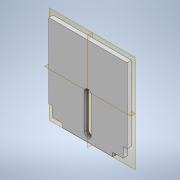
# Autodesk Inventor part: Hammer_wall
Saved by Autodesk Inventor 2021 (Build 250183000, 183)
## iProperties
Created: 2021-02-17
Part Number: Hammer_wall
Material: Generic
Document SubType Name: Modeling
Designer: negt20
Density: 1 g/cm^3
Appearance: Default
Author: negt20
Autodesk Inventor part; units mm, degrees
sketch "Sketch1" plane through (0, 0, 0) normal (0, 0, 1) x (1, 0, 0)
  line L0 (-55.5, 62.75) -> (55.5, 62.75)
  line L1 (55.5, 62.75) -> (55.5, -62.75)
  line L2 (55.5, -62.75) -> (-55.5, -62.75)
  line L3 (-55.5, -62.75) -> (-55.5, 62.75)
  point P0 (0, 62.75)
  point P1 (0, 0)
  point P2 (-55.5, 0)
  dimension "d0" = 111
  dimension "d1" = 125.5
  constraints: 8 end point, 2 midpoint, 2 parallel, 1 horizontal, 1 horizontal alignment, 1 perpendicular, 1 vertical alignment
  measures "d0" distance of L1.end L2.end
  measures "d1" distance of L0.end L1.end
extrude "Extrusion1" add sketch "Sketch1" along normal blind 6
sketch "Sketch2" plane through (0, 0, 6) normal (0, 0, 1) x (1, 0, 0)
  line L0 (-55.5, 62.75) -> (-55.5, -62.75) projected
  line L1 (-55.5, -62.75) -> (-55.5, -42.75)
  line L2 (-55.5, -42.75) -> (-50, -42.75)
  line L3 (-50, -42.75) -> (-50, -57.25)
  line L4 (-50, -57.25) -> (-35.5, -57.25)
  line L5 (-35.5, -57.25) -> (-35.5, -62.75)
  line L6 (-55.5, -62.75) -> (55.5, -62.75) projected
  line L7 (-35.5, -62.75) -> (-55.5, -62.75)
  point P0 (0, 0)
  point P1 (55.5, -62.75)
  point P2 (40.5, -62.5)
  dimension "d14" = 20
  dimension "d15" = 5.5
  dimension "d16" = 14.5
  dimension "d17" = 14.5
  constraints: 12 end point, 5 perpendicular, 1 point on line, 2 other
  measures "d14" distance of L0.end L1.end
  measures "d15" distance of L1.end L2.end
  measures "d16" distance of L2.end L3.end
  measures "d17" distance of L3.end L4.end
extrude "Extrusion2" cut sketch "Sketch2" against normal blind 15
mirror "Mirror1" about plane through (0, 0, 0) normal (1, 0, 0) of "Extrusion2"
sketch "Sketch3" plane through (0, 0, 6) normal (0, 0, 1) x (1, 0, 0)
  line L0 (-55.5, -62.75) -> (55.5, -62.75) projected
  line L1 (0, -62.75) -> (0, -52.25) construction
  line L2 (-5, -2.25) -> (5, -2.25) construction
  line L3 (5, -2.25) -> (5, -52.25)
  line L4 (5, -52.25) -> (-5, -52.25) construction
  line L5 (-5, -52.25) -> (-5, -2.25)
  arc A0 (5, -2.25) -> (-5, -2.25) centre (0, -2.25) ccw
  arc A1 (-5, -52.25) -> (5, -52.25) centre (0, -52.25) ccw
  point P0 (0, 0)
  point P1 (-40.5, -62.5)
  point P2 (40.5, -62.5)
  dimension "d9" = 10.5
  dimension "d10" = 10
  dimension "d11" = 50
  constraints: 10 end point, 4 point on circle, 3 coincident, 2 centre point, 2 midpoint, 2 parallel, 1 horizontal, 1 perpendicular, 1 vertical, 2 other
  measures "d9" distance of L1.start L1.end
  measures "d10" distance of L3.end L4.end
  measures "d11" distance of L2.end L3.end
extrude "Extrusion3" cut sketch "Sketch3" against normal blind 6
equation "\"d7\" = d5"
equation "\"d5\" = 15"
body "Solid1"
